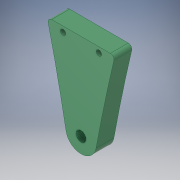
# Autodesk Inventor part: joint3_rot
Saved by Autodesk Inventor 2019 (Build 230136000, 136)
## iProperties
Created: 2019-12-29
Part Number: joint3_rot
Material: Пластик АБС
Document SubType Name: Modeling
Designer: Петров Иван
Density: 1.06 g/cm^3
Appearance: Гладкий — темный цвет морской волны
Author: Петров Иван
Autodesk Inventor part; units mm, degrees
ref_plane "YZ Plane" through (0, 0, 0) normal (1, 0, 0) x (0, 1, 0)
ref_plane "XZ Plane" through (0, 0, 0) normal (0, 1, 0) x (-1, 0, 0)
ref_plane "XY Plane" through (0, 0, 0) normal (0, 0, 1) x (1, 0, 0)
sketch "Эскиз1" plane through (0, 0, 0) normal (0, 0, 1) x (1, 0, 0)
  circle A0 centre (0, 0) radius 3.9
  line L0 (-3.9, 0) -> (-3.9, 42.320681)
  line L1 (3.9, 42.320681) -> (3.9, 0)
  arc A1 (3.9, 42.320681) -> (-3.9, 42.320681) centre (0, 0) ccw
  line L2 (-3.9, 42.320681) -> (-3.9, 48.320681)
  line L3 (-3.9, 48.320681) -> (3.9, 48.320681)
  line L4 (3.9, 48.320681) -> (3.9, 42.320681)
  circle A2 centre (0, 0) radius 7.5
  point P0 (0, 0)
  point P1 (0, -39)
  dimension "d0" = 0
  dimension "d1" = 6
  dimension "d2" = 15
  constraints: 10 end point, 4 point on circle, 3 centre point, 2 perpendicular, 2 vertical, 1 coincident, 1 parallel, 1 tangent
  measures "d0" distance of A0.centre A1.centre
  measures "d1" distance of L0.end L2.end
  measures "d2" diameter of A2
extrude "Выдавливание1" add sketch "Эскиз1" along normal blind 10 contours L1 A2 L0 A0 | A0 L0 A2 L1 | A2 L0 A1 L1 | A1 L2 L3 L4
sketch "Эскиз3" plane through (0, 0, 10) normal (0, 0, 1) x (1, 0, 0)
  line L0 (3.9, 48.320681) -> (-3.9, 48.320681)
  line L1 (-3.9, 48.320681) -> (-18.9, 48.320681)
  line L2 (-18.9, 48.320681) -> (-7.5, 0)
  arc A0 (-3.9, 6.406247) -> (3.9, 6.406247) centre (0, 0) ccw
  line L3 (3.9, 6.406247) -> (3.9, 48.320681)
  line L4 (3.9, 48.320681) -> (18.9, 48.320681)
  line L5 (18.9, 48.320681) -> (7.5, 0)
  arc A1 (7.5, 0) -> (-7.5, 0) centre (0, 0) ccw
  line L6 (-3.9, 48.320681) -> (-3.9, 43.72824)
  line L7 (-3.9, 43.72824) -> (3.9, 43.72824)
  line L8 (3.9, 48.320681) -> (3.9, 43.72824)
  point P0 (0, 0)
  dimension "d13" = 15
  dimension "d14" = 15
  constraints: 14 end point, 4 point on circle, 2 horizontal, 1 centre point, 1 collinear, 1 concentric, 1 perpendicular, 1 point on line, 1 vertical
  measures "d13" distance of L0.end L1.end
  measures "d14" distance of L0.start L4.end
extrude "Выдавливание3" add sketch "Эскиз3" against normal blind 10 contours L4 L5 A0 L3 | L6 L7 L3 A1 A0 L2 L1
sketch "Эскиз4" plane through (0, 0, 10) normal (0, 0, 1) x (1, 0, 0)
  line L0 (18.9, 48.320681) -> (-18.9, 48.320681)
  line L1 (0, 48.320681) -> (0, 45.320681)
  line L2 (0, 45.320681) -> (-10, 45.320681)
  line L3 (-10, 45.320681) -> (10, 45.320681)
  circle A0 centre (-10, 45.320681) radius 1.5
  circle A1 centre (10, 45.320681) radius 1.5
  point P0 (0, 0)
  dimension "d17" = 3
  dimension "d18" = 10
  dimension "d19" = 20
  dimension "d20" = 3
  dimension "d21" = 3
  constraints: 6 end point, 2 centre point, 2 coincident, 1 midpoint, 1 perpendicular, 1 point on line, 1 vertical
  measures "d17" distance of L1.start L1.end
  measures "d18" distance of L1.end L2.end
  measures "d19" distance of L2.end L3.end
  measures "d20" diameter of A0
  measures "d21" diameter of A1
extrude "Выдавливание4" cut sketch "Эскиз4" against normal blind 10
thicken "Толщина2" operation add thickness 1 both sides no extend neighbours yes toward (-0.9870503, -0.1604113, 0) faces at (-7.402877, -1.203085, 3.333333)
sketch "Эскиз5" plane through (0, 0, 10) normal (0, 0, 1) x (1, 0, 0)
  line L0 (2.87853, -0.352228) -> (2.533905, -0.473669)
  arc A0 (2.87853, -0.352228) -> (2.894239, -0.182698) centre (0, 0) ccw
  line L1 (2.577797, 0) -> (2.894239, -0.182698)
  line L2 (2.894239, 0.182698) -> (2.577797, 0)
  arc A1 (2.894239, 0.182698) -> (2.87853, 0.352228) centre (0, 0) ccw
  line L3 (2.533905, 0.473669) -> (2.87853, 0.352228)
  line L4 (2.811389, 0.711402) -> (2.533905, 0.473669)
  arc A2 (2.811389, 0.711402) -> (2.764796, 0.875159) centre (0, 0) ccw
  line L5 (2.403724, 0.931208) -> (2.764796, 0.875159)
  line L6 (2.6328, 1.215881) -> (2.403724, 0.931208)
  arc A3 (2.6328, 1.215881) -> (2.55691, 1.368288) centre (0, 0) ccw
  line L7 (2.191687, 1.357035) -> (2.55691, 1.368288)
  line L8 (2.364554, 1.678954) -> (2.191687, 1.357035)
  arc A4 (2.364554, 1.678954) -> (2.261952, 1.814821) centre (0, 0) ccw
  line L9 (1.905015, 1.73665) -> (2.261952, 1.814821)
  line L10 (2.015786, 2.084852) -> (1.905015, 1.73665)
  arc A5 (2.015786, 2.084852) -> (1.889965, 2.199553) centre (0, 0) ccw
  line L11 (1.55347, 2.057126) -> (1.889965, 2.199553)
  line L12 (1.598373, 2.419753) -> (1.55347, 2.057126)
  arc A6 (1.598373, 2.419753) -> (1.453618, 2.509381) centre (0, 0) ccw
  line L13 (1.149023, 2.307549) -> (1.453618, 2.509381)
  line L14 (1.126529, 2.672252) -> (1.149023, 2.307549)
  arc A7 (1.126529, 2.672252) -> (0.96777, 2.733756) centre (0, 0) ccw
  line L15 (0.705448, 2.479391) -> (0.96777, 2.733756)
  line L16 (0.616322, 2.833751) -> (0.705448, 2.479391)
  arc A8 (0.616322, 2.833751) -> (0.448966, 2.865036) centre (0, 0) ccw
  line L17 (0.237849, 2.5668) -> (0.448966, 2.865036)
  line L18 (0.085128, 2.89875) -> (0.237849, 2.5668)
  arc A9 (0.085128, 2.89875) -> (-0.085128, 2.89875) centre (0, 0) ccw
  line L19 (-0.237849, 2.5668) -> (-0.085128, 2.89875)
  line L20 (-0.448966, 2.865036) -> (-0.237849, 2.5668)
  arc A10 (-0.448966, 2.865036) -> (-0.616322, 2.833751) centre (0, 0) ccw
  line L21 (-0.705448, 2.479391) -> (-0.616322, 2.833751)
  line L22 (-0.96777, 2.733756) -> (-0.705448, 2.479391)
  arc A11 (-0.96777, 2.733756) -> (-1.126529, 2.672252) centre (0, 0) ccw
  line L23 (-1.149023, 2.307549) -> (-1.126529, 2.672252)
  line L24 (-1.453618, 2.509381) -> (-1.149023, 2.307549)
  arc A12 (-1.453618, 2.509381) -> (-1.598373, 2.419753) centre (0, 0) ccw
  line L25 (-1.55347, 2.057126) -> (-1.598373, 2.419753)
  line L26 (-1.889965, 2.199553) -> (-1.55347, 2.057126)
  arc A13 (-1.889965, 2.199553) -> (-2.015786, 2.084852) centre (0, 0) ccw
  line L27 (-1.905015, 1.73665) -> (-2.015786, 2.084852)
  line L28 (-2.261952, 1.814821) -> (-1.905015, 1.73665)
  arc A14 (-2.261952, 1.814821) -> (-2.364554, 1.678954) centre (0, 0) ccw
  line L29 (-2.191687, 1.357035) -> (-2.364554, 1.678954)
  line L30 (-2.55691, 1.368288) -> (-2.191687, 1.357035)
  arc A15 (-2.55691, 1.368288) -> (-2.6328, 1.215881) centre (0, 0) ccw
  line L31 (-2.403724, 0.931208) -> (-2.6328, 1.215881)
  line L32 (-2.764796, 0.875159) -> (-2.403724, 0.931208)
  arc A16 (-2.764796, 0.875159) -> (-2.811389, 0.711402) centre (0, 0) ccw
  line L33 (-2.533905, 0.473669) -> (-2.811389, 0.711402)
  line L34 (-2.87853, 0.352228) -> (-2.533905, 0.473669)
  arc A17 (-2.87853, 0.352228) -> (-2.894239, 0.182698) centre (0, 0) ccw
  line L35 (-2.577797, 0) -> (-2.894239, 0.182698)
  line L36 (-2.894239, -0.182698) -> (-2.577797, 0)
  arc A18 (-2.894239, -0.182698) -> (-2.87853, -0.352228) centre (0, 0) ccw
  line L37 (-2.533905, -0.473669) -> (-2.87853, -0.352228)
  line L38 (-2.811389, -0.711402) -> (-2.533905, -0.473669)
  arc A19 (-2.811389, -0.711402) -> (-2.764796, -0.875159) centre (0, 0) ccw
  line L39 (-2.403724, -0.931208) -> (-2.764796, -0.875159)
  line L40 (-2.6328, -1.215881) -> (-2.403724, -0.931208)
  arc A20 (-2.6328, -1.215881) -> (-2.55691, -1.368288) centre (0, 0) ccw
  line L41 (-2.191687, -1.357035) -> (-2.55691, -1.368288)
  line L42 (-2.364554, -1.678954) -> (-2.191687, -1.357035)
  arc A21 (-2.364554, -1.678954) -> (-2.261952, -1.814821) centre (0, 0) ccw
  line L43 (-1.905015, -1.73665) -> (-2.261952, -1.814821)
  line L44 (-2.015786, -2.084852) -> (-1.905015, -1.73665)
  arc A22 (-2.015786, -2.084852) -> (-1.889965, -2.199553) centre (0, 0) ccw
  line L45 (-1.55347, -2.057126) -> (-1.889965, -2.199553)
  line L46 (-1.598373, -2.419753) -> (-1.55347, -2.057126)
  arc A23 (-1.598373, -2.419753) -> (-1.453618, -2.509381) centre (0, 0) ccw
  line L47 (-1.149023, -2.307549) -> (-1.453618, -2.509381)
  line L48 (-1.126529, -2.672252) -> (-1.149023, -2.307549)
  arc A24 (-1.126529, -2.672252) -> (-0.96777, -2.733756) centre (0, 0) ccw
  line L49 (-0.705448, -2.479391) -> (-0.96777, -2.733756)
  line L50 (-0.616322, -2.833751) -> (-0.705448, -2.479391)
  arc A25 (-0.616322, -2.833751) -> (-0.448966, -2.865036) centre (0, 0) ccw
  line L51 (-0.237849, -2.5668) -> (-0.448966, -2.865036)
  line L52 (-0.085128, -2.89875) -> (-0.237849, -2.5668)
  arc A26 (-0.085128, -2.89875) -> (0.085128, -2.89875) centre (0, 0) ccw
  line L53 (0.237849, -2.5668) -> (0.085128, -2.89875)
  line L54 (0.448966, -2.865036) -> (0.237849, -2.5668)
  arc A27 (0.448966, -2.865036) -> (0.616322, -2.833751) centre (0, 0) ccw
  line L55 (0.705448, -2.479391) -> (0.616322, -2.833751)
  line L56 (0.96777, -2.733756) -> (0.705448, -2.479391)
  arc A28 (0.96777, -2.733756) -> (1.126529, -2.672252) centre (0, 0) ccw
  line L57 (1.149023, -2.307549) -> (1.126529, -2.672252)
  line L58 (1.453618, -2.509381) -> (1.149023, -2.307549)
  arc A29 (1.453618, -2.509381) -> (1.598373, -2.419753) centre (0, 0) ccw
  line L59 (1.55347, -2.057126) -> (1.598373, -2.419753)
  line L60 (1.889965, -2.199553) -> (1.55347, -2.057126)
  arc A30 (1.889965, -2.199553) -> (2.015786, -2.084852) centre (0, 0) ccw
  line L61 (1.905015, -1.73665) -> (2.015786, -2.084852)
  line L62 (2.261952, -1.814821) -> (1.905015, -1.73665)
  arc A31 (2.261952, -1.814821) -> (2.364554, -1.678954) centre (0, 0) ccw
  line L63 (2.191687, -1.357035) -> (2.364554, -1.678954)
  line L64 (2.55691, -1.368288) -> (2.191687, -1.357035)
  arc A32 (2.55691, -1.368288) -> (2.6328, -1.215881) centre (0, 0) ccw
  line L65 (2.403724, -0.931208) -> (2.6328, -1.215881)
  line L66 (2.764796, -0.875159) -> (2.403724, -0.931208)
  arc A33 (2.764796, -0.875159) -> (2.811389, -0.711402) centre (0, 0) ccw
  line L67 (2.533905, -0.473669) -> (2.811389, -0.711402)
  circle A34 centre (0, 0) radius 2.4
  circle A35 centre (0, 0) radius 2.4
  circle A36 centre (0, 0) radius 1.25
  circle A37 centre (0, 0) radius 3.9
  point P0 (-10.35, -10)
  constraints: 136 end point, 68 point on circle, 38 centre point, 1 coincident
extrude "Выдавливание5" add sketch "Эскиз5" against normal up to surface (10 mm away) contours A37
fillet "Сопряжение3" radius 2 2 edges at (18.9, 48.3207, 5) (-18.9, 48.3207, 5)
fillet "Сопряжение4" radius 996.5 2 edges at (8.1045, 2.5625, 5) (-8.1045, 2.5625, 5)
equation "\"d14\" = d13"
